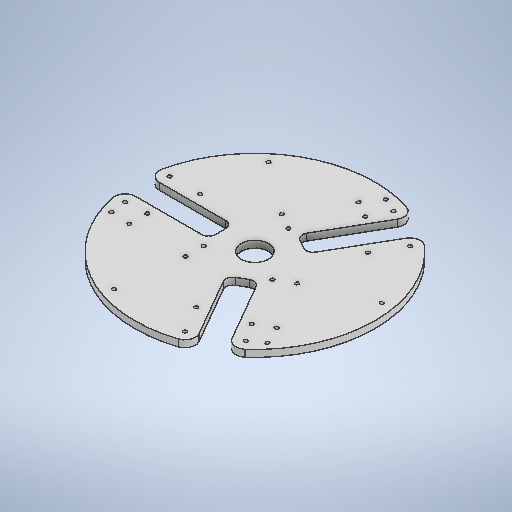
# Autodesk Inventor part: RT_FRM_V2_MC_004_BottomDynamicsPlate
Saved by Autodesk Inventor 2025.3 (Build 293356000, 356)
## iProperties
Created: 2026-04-28
Part Number: RT_FRM_V2_MC_004_BottomDynamicsPlate
Material: Generic
Document SubType Name: Modeling
Designer: louis
Density: 1 g/cm^3
Appearance: Default
Mass: 556.266 g
Surface Area: 1307.88 cm^2
Volume: 556.266 cm^3
Author: louis
Autodesk Inventor part; units mm, degrees
ref_plane "YZ Plane" through (0, 0, 0) normal (1, 0, 0) x (0, 1, 0)
ref_plane "XZ Plane" through (0, 0, 0) normal (0, 1, 0) x (-1, 0, 0)
ref_plane "XY Plane" through (0, 0, 0) normal (0, 0, 1) x (1, 0, 0)
sketch "Sketch1" plane through (0, 0, 0) normal (0, 1, 0) x (-1, 0, 0)
  line L0 (30, -2.5) -> (140, -2.5)
  line L1 (145, 0) -> (25, 0)
  line L2 (0, 0) -> (25, 0)
  circle A0 centre (0, 0) radius 175
  line L3 (50, 0) -> (103.8137, 0) construction
  line L4 (135, 16.5) -> (35, 16.5)
  line L5 (35, 16.5) -> (35, 66.5)
  line L6 (35, 66.5) -> (135, 66.5)
  line L7 (135, 66.5) -> (135, 16.5)
  line L8 (85, 16.5) -> (85, 0) construction
  line L9 (85, 66.5) -> (85, 16.5) construction
  line L10 (126, 30.5) -> (85, 30.5) construction
  line L11 (126, 30.5) -> (126, 57) construction
  line L12 (174.1228, -17.5) -> (50, -17.5)
  line L13 (50, -17.5) -> (50, 17.5)
  line L14 (50, 17.5) -> (174.1228, 17.5)
  line L15 (174.1228, 17.5) -> (174.1228, -17.5)
  line L16 (0, 0) -> (0, 175)
  line L17 (160, 17.5) -> (160, 117.5)
  line L18 (160, 117.5) -> (-67.8387, 117.5)
  line L19 (-67.8387, 117.5) -> (0, 0)
  circle A1 centre (0, 0) radius 310 construction
  line L20 (-310, -390) -> (-310, -310) construction
  line L21 (-310, -310) -> (-390, -310) construction
  line L22 (-390, -310) -> (-390, -390) construction
  line L23 (-390, -390) -> (-310, -390) construction
  line L24 (-310, -390) -> (-390, -310) construction
  line L25 (-310, -310) -> (-390, -390) construction
  line L26 (-310, 310) -> (-310, 390) construction
  line L27 (-310, 390) -> (-390, 390) construction
  line L28 (-390, 390) -> (-390, 310) construction
  line L29 (-390, 310) -> (-310, 310) construction
  line L30 (-310, 310) -> (-390, 390) construction
  line L31 (-310, 390) -> (-390, 310) construction
  line L32 (390, 310) -> (390, 390) construction
  line L33 (390, 390) -> (310, 390) construction
  line L34 (310, 390) -> (310, 310) construction
  line L35 (310, 310) -> (390, 310) construction
  line L36 (390, 310) -> (310, 390) construction
  line L37 (390, 390) -> (310, 310) construction
  line L38 (390, -390) -> (390, -310) construction
  line L39 (390, -310) -> (310, -310) construction
  line L40 (310, -310) -> (310, -390) construction
  line L41 (310, -390) -> (390, -390) construction
  line L42 (390, -390) -> (310, -310) construction
  line L43 (390, -310) -> (310, -390) construction
  line L44 (310, -310) -> (310, 310) construction
  line L45 (310, 310) -> (-310, 310) construction
  line L46 (-310, 310) -> (-310, -310) construction
  line L47 (-310, -310) -> (310, -310) construction
  line L48 (-67.8387, 117.5) -> (-87.5, 151.5544)
  line L49 (160, 17.5) -> (174.1228, 17.5)
  line L50 (-102.2168, 142.0448) -> (-71.906, 159.5448)
  line L51 (-71.906, -159.5448) -> (-102.2168, -142.0448)
  point P0 (44, 30.5)
  point P1 (44, 57)
  point P2 (161.4582, -67.5)
  point P3 (50, 0)
  point P4 (-71.906, 159.5448)
  point P5 (-87.0614, 150.7948)
  point P6 (-102.2168, 142.0448)
  point P7 (160, 70.8872)
  point P8 (129.6871, 117.5)
  point P9 (0, 117.5)
  dimension "d0" = 110
  dimension "d2" = 2.5
  dimension "d4" = 85
  dimension "d9" = 350
  dimension "d11" = 19
  dimension "d12" = 50
  dimension "d13" = 100
  dimension "d14" = 26.5
  dimension "d15" = 82
  dimension "d26" = 35
  dimension "d27" = 35
  dimension "d33" = 9.5
  dimension "d40" = 50
  dimension "d46" = 120
  dimension "d47" = 100
  dimension "d48" = 25
  dimension "d74" = 80
  dimension "d75" = 80
  dimension "d78" = 80
  dimension "d79" = 80
  dimension "d80" = 80
  dimension "d81" = 80
  dimension "d82" = 80
  dimension "d83" = 80
  dimension "d86" = 620
  dimension "d97" = 360
  constraints: 104 end point, 14 perpendicular, 12 parallel, 7 vertical, 5 point on circle, 4 horizontal, 4 point on line, 3 coincident, 3 midpoint, 3 tangent, 2 centre point, 2 collinear, 2 symmetric about line, 10 other
  measures "d0" distance of L0.end L0.start
  measures "d2" distance between parallel lines of L0 L1
  measures "d4" distance of L2.start L8.end
  measures "d9" diameter of A0
  measures "d11" distance from line of L0 L4.start
  measures "d12" distance of L6.end L4.start
  measures "d13" distance of L4.start L4.end
  measures "d14" distance of L11.end L10.start
  measures "d15" distance of L10.start point (44, 30.5)
  measures "d26" distance between parallel lines of L14 L12
  measures "d27" distance between parallel lines of L8 L13
  measures "d33" distance from line of L6 L11.end
  measures "d40" distance from line of L12 point (161.458, -67.5)
  measures "d46" angle of L19 L2
  measures "d47" distance of L17.start L17.end
  measures "d48" distance between parallel lines of L17 L7
  measures "d74" distance of L21.end L22.end
  measures "d75" distance of L22.end L20.start
  measures "d78" distance of L27.end L28.end
  measures "d79" distance of L28.end L26.start
  measures "d80" distance of L33.end L34.end
  measures "d81" distance of L34.end L32.start
  measures "d82" distance of L39.end L40.end
  measures "d83" distance of L40.end L38.start
  measures "d86" distance of L34.end L26.start
extrude "Extrusion1" add sketch "Sketch1" against normal blind 10 contours L1 L2 L16 L18 A0 L17 L14 L7 L6 L5 L4 L13 | L4 L5 L6 L7 L14 L13 | L19 L18 L16 | L18 L48 L50 A0 L16 | L16 A0 L18 | L14 L17 A0
pattern_circular "Circular Pattern2" count 3 over 360 about axis through (0, 0, 0) along (0, -1, 0) of "Extrusion1"
hole "Hole1" at (-126, 0, 30.5) at (-44, 0, 30.5) at (-126, 0, 57) at (-44, 0, 57) direction (0, -1, 0) diameter 5.5 end through all counterbore diameter 10 counterbore depth 5 clearance for "Socket Head Cap Screw" size "M5" standard "Ansi Metric M Profile"
extrude "Extrusion2" cut sketch "Sketch1" against normal blind 10 contours L13 L4 L7 L14 L15 L12 | L13 L14 L7 L4
pattern_circular "Circular Pattern1" count 3 over 360 about axis through (0, -10, 0) along (0, 1, 0) of "Hole1", "Extrusion2"
fillet "Fillet1" radius 10 6 edges at (9.8446, -5, 52.0513) (40.1554, -5, -34.5513) (-50, -5, -17.5) (-50, -5, 17.5) (40.1554, -5, 34.5513) (9.8446, -5, -52.0513)
sketch "Sketch3" plane through (0, -10, 0) normal (0, -1, 0) x (1, 0, 0)
  arc A0 (71.906, 159.5448) -> (-174.1228, 17.5) centre (0, 0) ccw projected
  line L0 (0, 0) -> (-392.8558, 0)
  line L1 (0, 0) -> (87.5, 151.5544)
  circle A1 centre (0, 0) radius 20
  arc A2 (102.2168, -142.0448) -> (102.2168, 142.0448) centre (0, 0) ccw projected
  line L2 (-35.75, 35.75) -> (35.75, 35.75) construction
  line L3 (35.75, 35.75) -> (35.75, -35.75) construction
  line L4 (35.75, -35.75) -> (-35.75, -35.75) construction
  line L5 (-35.75, -35.75) -> (-35.75, 35.75) construction
  line L6 (-35.75, 35.75) -> (35.75, -35.75) construction
  line L7 (35.75, 35.75) -> (-35.75, -35.75) construction
  point P0 (141.3901, 103.1204)
  point P1 (100.1684, 143.4967)
  dimension "d99" = 120
  dimension "d100" = 40
  dimension "d101" = 71.5
  dimension "d102" = 71.5
  constraints: 16 end point, 2 horizontal, 2 midpoint, 2 parallel, 1 centre point, 1 coincident, 1 perpendicular, 1 point on circle
  measures "d99" angle of L0 L1
  measures "d100" diameter of A1
  measures "d101" distance of L3.end L4.end
  measures "d102" distance of L2.end L3.end
extrude "Extrusion3" cut sketch "Sketch3" against normal up to surface (10 mm away)
fillet "Fillet2" radius 15 6 edges at (-174.1228, -5, 17.5) (-174.1228, -5, -17.5) (102.2168, -5, -142.0448) (102.2168, -5, 142.0448) (71.906, -5, 159.5448) (71.906, -5, -159.5448)
sketch "Sketch4" plane through (0, 0, 0) normal (0, 1, 0) x (1, 0, 0)
  circle A0 centre (377.3654, 14.0861) radius 175
  arc A1 (440.5422, 158.5115) -> (432.2568, 180.2545) centre (427.5518, 166.0115) ccw
  circle A2 centre (427.5518, 166.0115) radius 15
  arc A3 (432.2568, 180.2545) -> (206.0137, 49.633) centre (377.3654, 14.0861) ccw
  line L0 (402.21, 92.1181) -> (440.5422, 158.5115)
  circle A4 centre (377.3654, 14.0861) radius 3.3
  circle A5 centre (377.3654, 14.0861) radius 60
  line L1 (440.5422, 158.5115) -> (390.9056, 72.5383)
  line L2 (307.3654, 6.5861) -> (307.3654, 21.5861)
  line L3 (307.3654, 14.0861) -> (307.3654, 174.4762)
  circle A6 centre (322.3654, 65.0763) radius 15
  circle A7 centre (383.0159, 88.8729) radius 15
  circle A8 centre (322.3654, 164.3359) radius 15
  line L4 (427.5518, 166.0115) -> (322.3654, 164.3359) construction
  line L5 (322.3654, 164.3359) -> (322.3654, 65.0763) construction
  line L6 (322.3654, 65.0763) -> (383.0159, 88.8729) construction
  line L7 (383.0159, 88.8729) -> (427.5518, 166.0115) construction
  arc A9 (427.5518, 166.0115) -> (322.3654, 164.3359) centre (377.4076, 11.4417) ccw construction
  line L8 (297.3654, 31.5861) -> (220.701, 31.5861)
  line L9 (235.701, 31.5861) -> (235.701, 116.8294)
  arc A10 (206.0137, 49.633) -> (220.701, 31.5861) centre (220.701, 46.5861) ccw
  arc A11 (220.701, 31.5861) -> (230.701, 41.5861) centre (220.701, 41.5861) ccw
  line L10 (230.701, 41.5861) -> (230.701, 109.5562)
  circle A12 centre (225.701, 90.8838) radius 5
  arc A13 (432.2568, 180.2545) -> (206.0137, 49.633) centre (377.3654, 14.0861) ccw
  line L11 (220.701, 46.5861) -> (225.701, 90.8838) construction
  arc A14 (-156.6645, -17.5) -> (-171.3517, -35.5469) centre (-156.6645, -32.5) ccw projected
  arc A15 (-171.3517, -35.5469) -> (54.8914, -166.1684) centre (0, 0) ccw projected
  arc A16 (-146.6645, -27.5) -> (-156.6645, -17.5) centre (-156.6645, -27.5) ccw
  line L12 (-146.6645, -27.5) -> (-146.6645, -95.4701)
  circle A17 centre (-151.6645, -76.7978) radius 5
  circle A18 centre (0, 0) radius 20 projected
  circle A19 centre (0, 0) radius 60
  line L13 (-70, -160.3901) -> (-70, 0)
  arc A20 (54.8914, -166.1684) -> (63.1768, -144.4254) centre (50.1864, -151.9254) ccw projected
  line L14 (63.1768, -144.4254) -> (14.8446, -60.7115) projected
  circle A21 centre (-55, -50.9902) radius 15
  circle A22 centre (-55, -150.2498) radius 15
  circle A23 centre (5.6504, -74.7868) radius 15
  line L15 (5.6504, -74.7868) -> (-55, -50.9902) construction
  line L16 (-55, -50.9902) -> (-55, -150.2498) construction
  line L17 (-55, -150.2498) -> (50.1864, -151.9254) construction
  line L18 (50.1864, -151.9254) -> (5.6504, -74.7868) construction
  circle A24 centre (0, 0) radius 160 construction
  line L19 (-2.4068, -151.0876) -> (-2.5485, -159.9797) construction
  line L20 (-156.6645, -32.5) -> (-151.6645, -76.7978) construction
  point P0 (374.8193, 173.9211)
  point P1 (352.6907, 76.9746)
  point P2 (405.2839, 127.4422)
  point P3 (322.3654, 114.7061)
  point P4 (223.201, 68.735)
  point P5 (-55, -150.2498)
  point P6 (27.9184, -113.3561)
  point P7 (-55, -100.62)
  point P8 (-24.6748, -62.8885)
  point P9 (-154.1645, -54.6489)
  dimension "d114" = 120
  dimension "d113" = 350
  dimension "d115" = 30
  dimension "d116" = 30
  dimension "d117" = 30
  dimension "d118" = 162.5
  dimension "d119" = 10
  dimension "d120" = 10
  dimension "d125" = 10
  dimension "d126" = 10
  dimension "d127" = 120
  dimension "d128" = 70
  dimension "d129" = 30
  dimension "d131" = 30
  dimension "d132" = 30
  constraints: 40 end point, 23 point on circle, 19 centre point, 18 tangent, 16 coincident, 11 midpoint, 3 vertical, 2 perpendicular, 2 point on line, 1 parallel, 10 other
  measures "d113" diameter of A0
  measures "d115" diameter of A6
  measures "d116" diameter of A7
  measures "d117" diameter of A8
  measures "d118" radius of A9
  measures "d119" radius of A11
  measures "d120" diameter of A12
  measures "d125" radius of A16
  measures "d126" diameter of A17
  measures "d127" diameter of A19
  measures "d128" distance from line of A15.centre L13
  measures "d129" diameter of A21
  measures "d131" diameter of A22
  measures "d132" diameter of A23
hole "Hole4" at (352.6907, 0, -76.9746) at (322.3654, 0, -114.7061) at (405.2839, 0, -127.4422) at (427.5518, 0, -166.0115) at (322.3654, 0, -164.3359) at (374.8193, 0, -173.9211) at (220.701, 0, -46.5861) at (223.201, 0, -68.735) at (322.3654, 0, -65.0763) at (383.0159, 0, -88.8729) at (-55, 0, 150.2498) at (50.1864, 0, 151.9254) at (27.9184, 0, 113.3561) at (-154.1645, 0, 54.6489) at (-156.6645, 0, 32.5) direction (0, -1, 0) diameter 5.5 end through all start extended yes countersink diameter 10.4 countersink angle 90 clearance for "Flat Head Machine Screw" size "M5" standard "Ansi Metric M Profile"
pattern_circular "Circular Pattern4" count 3 over 360 about axis through (0, -10, 0) along (0, 1, 0) of "Hole4"
mirror "Mirror1" about plane through (0, 0, 0) normal (0, 1, 0) remove original yes
body "Solid1"
